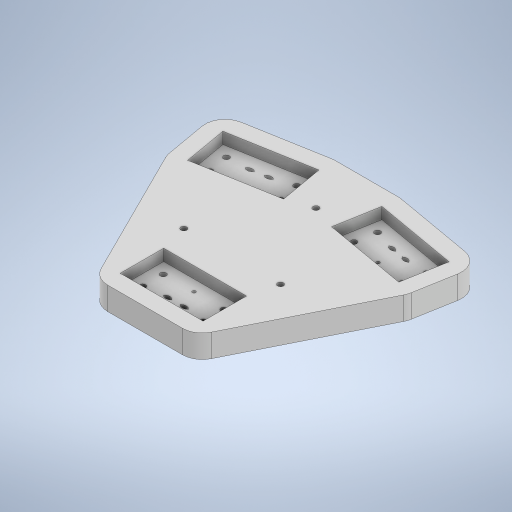
# Autodesk Inventor part: Baseplate
Saved by Autodesk Inventor 2023 (Build 270158000, 158)
## iProperties
Created: 2023-07-20
Part Number: Baseplate
Material: Generic
Document SubType Name: Modeling
Designer: campstudent
Density: 1 g/cm^3
Appearance: Default
Author: campstudent
Autodesk Inventor part; units mm, degrees
ref_plane "YZ Plane" through (0, 0, 0) normal (1, 0, 0) x (0, 1, 0)
ref_plane "XZ Plane" through (0, 0, 0) normal (0, 1, 0) x (-1, 0, 0)
ref_plane "XY Plane" through (0, 0, 0) normal (0, 0, 1) x (1, 0, 0)
sketch "Sketch1" plane through (0, 0, 0) normal (0, 1, 0) x (-1, 0, 0)
  line L0 (0, 0) -> (-160, 0)
  line L1 (-160, 0) -> (-160, -160)
  line L2 (-160, -160) -> (0, -160)
  line L3 (0, -160) -> (0, 0)
  dimension "d0" = 160
  dimension "d1" = 160
  constraints: 8 end point, 2 parallel, 1 horizontal, 1 perpendicular
  measures "d0" distance of L2.end L0.start
  measures "d1" distance of L0.end L0.start
extrude "Extrusion1" add sketch "Sketch1" along normal blind 14
sketch "Sketch2" plane through (0, 14, 0) normal (0, 1, 0) x (1, 0, 0)
  line L0 (54.75, 30) -> (105.25, 30)
  line L1 (105.25, 30) -> (105.25, 56.5)
  line L2 (105.25, 56.5) -> (54.75, 56.5)
  line L3 (54.75, 56.5) -> (54.75, 30)
  line L4 (0, 0) -> (160, 0) projected
  line L5 (0, 160) -> (0, 0) projected
  line L6 (11.0918, 136.251) -> (15.6934, 110.1536)
  line L7 (15.6934, 110.1536) -> (65.4262, 118.9228)
  line L8 (65.4262, 118.9228) -> (60.8246, 145.0203)
  line L9 (60.8246, 145.0203) -> (11.0918, 136.251)
  line L10 (38.2588, 94.75) -> (38.2588, 145.25) construction
  line L11 (25.009, 127.5869) -> (51.509, 127.5869) construction
  line L12 (160, 160) -> (0, 160) projected
  line L13 (54.75, 43.25) -> (106.8484, 43.25) construction
  line L14 (80, 30) -> (80, 56.5) construction
  line L15 (80, 43.25) -> (80, 148.25)
  line L16 (148.9082, 136.251) -> (144.3066, 110.1536)
  line L17 (144.3066, 110.1536) -> (94.5738, 118.9228)
  line L18 (94.5738, 118.9228) -> (99.1754, 145.0203)
  line L19 (99.1754, 145.0203) -> (148.9082, 136.251)
  line L20 (98.0138, 136.2229) -> (145.4682, 118.9509) construction
  line L21 (126.2728, 140.0379) -> (117.2092, 115.136) construction
  line L22 (121.741, 127.5869) -> (85.8289, 28.9192)
  line L23 (38.259, 127.5869) -> (56.4995, 24.14) construction
  point P0 (38.2588, 120)
  point P1 (33.7272, 140.0379)
  point P2 (61.9862, 136.2229)
  dimension "d4" = 26.5
  dimension "d5" = 50.5
  dimension "d6" = 30
  dimension "d7" = 80
  dimension "d9" = 27.167
  dimension "d13" = 17.4333
  dimension "d15" = 12.4509
  dimension "d16" = 23.7272
  dimension "d17" = 11.0918
  dimension "d19" = 105
  dimension "d73" = 270
  constraints: 42 end point, 7 midpoint, 4 parallel, 2 equal length, 2 horizontal, 2 perpendicular, 2 point on line
  measures "d4" distance of L2.end L0.start
  measures "d5" distance of L0.start L0.end
  measures "d6" distance from line of L4 L0.start
  measures "d7" distance from line of L14.start L5
  measures "d9" horizontal distance of L6.start point (38.259, 120)
  measures "d13" vertical distance of L23.start L6.end
  measures "d15" vertical distance of L23.start point (33.727, 140.038)
  measures "d16" horizontal distance of point (61.986, 136.223) L23.start
  measures "d17" horizontal distance of L5.start L6.start
  measures "d19" distance of L15.start L15.end
extrude "Extrusion2" cut sketch "Sketch2" against normal blind 7
sketch "Sketch3" plane through (0, 7, 0) normal (0, 1, 0) x (1, 0, 0)
  circle A0 centre (21.1254, 118.2194) radius 1.8
  line L0 (11.0918, 136.251) -> (60.8246, 145.0203) construction
  line L1 (35.9582, 140.6356) -> (40.5598, 114.5382) construction
  line L2 (65.4262, 118.9228) -> (15.6934, 110.1536) construction
  circle A1 centre (18.9548, 130.5295) radius 1.8
  line L3 (15.6934, 110.1536) -> (11.0918, 136.251) projected
  circle A2 centre (57.5633, 124.6444) radius 1.8
  circle A3 centre (55.3926, 136.9545) radius 1.8
  line L4 (160, 160) -> (0, 160) construction
  line L5 (80, 160) -> (80, 0) construction
  line L6 (0, 0) -> (160, 0) construction
  circle A4 centre (138.8746, 118.2194) radius 1.8
  line L7 (124.0418, 140.6356) -> (119.4402, 114.5382) construction
  circle A5 centre (141.0452, 130.5295) radius 1.8
  circle A6 centre (102.4367, 124.6444) radius 1.8
  circle A7 centre (104.6074, 136.9545) radius 1.8
  circle A8 centre (61.5, 37) radius 1.8
  circle A9 centre (61.5, 49.5) radius 1.8
  line L8 (54.75, 56.5) -> (105.25, 56.5) projected
  line L9 (54.75, 30) -> (54.75, 56.5) projected
  line L10 (105.25, 30) -> (54.75, 30) projected
  circle A10 centre (98.5, 37) radius 1.8
  circle A11 centre (98.5, 49.5) radius 1.8
  circle A12 centre (120.6123, 121.1857) radius 1
  line L11 (144.3066, 110.1536) -> (94.5738, 118.9228) projected
  circle A13 centre (127.4464, 131.1503) radius 1.25
  line L12 (148.9082, 136.251) -> (144.3066, 110.1536) projected
  line L13 (127.4464, 131.1503) -> (129.9085, 130.7162) construction
  line L14 (129.9085, 130.7162) -> (124.9844, 131.5845) construction
  line L15 (99.1754, 145.0203) -> (148.9082, 136.251) construction
  arc A14 (129.9085, 130.7162) -> (124.9844, 131.5845) centre (127.1209, 129.3038) ccw
  arc A15 (124.9844, 131.5845) -> (129.9085, 130.7162) centre (127.772, 132.9968) ccw
  circle A16 centre (117.5984, 132.8868) radius 1.25
  line L16 (117.5984, 132.8868) -> (115.1364, 133.3209) construction
  line L17 (115.1364, 133.3209) -> (120.0604, 132.4527) construction
  arc A17 (120.0604, 132.4527) -> (115.1364, 133.3209) centre (117.2728, 131.0403) ccw
  arc A18 (115.1364, 133.3209) -> (120.0604, 132.4527) centre (117.924, 134.7333) ccw
  circle A19 centre (39.3877, 121.1857) radius 1
  circle A20 centre (32.5536, 131.1503) radius 1.25
  line L18 (32.5536, 131.1503) -> (30.0915, 130.7162) construction
  line L19 (30.0915, 130.7162) -> (35.0156, 131.5845) construction
  arc A21 (35.0156, 131.5845) -> (30.0915, 130.7162) centre (32.8791, 129.3038) ccw
  arc A22 (30.0915, 130.7162) -> (35.0156, 131.5845) centre (32.228, 132.9968) ccw
  line L20 (42.4016, 132.8868) -> (44.8636, 133.3209) construction
  circle A23 centre (42.4016, 132.8868) radius 1.25
  line L21 (44.8636, 133.3209) -> (39.9396, 132.4527) construction
  arc A24 (39.9396, 132.4527) -> (44.8636, 133.3209) centre (42.076, 134.7333) ccw
  arc A25 (44.8636, 133.3209) -> (39.9396, 132.4527) centre (42.7272, 131.0403) ccw
  circle A26 centre (80, 49.75) radius 1
  circle A27 centre (85, 38.75) radius 1.25
  line L22 (105.25, 56.5) -> (105.25, 30) projected
  line L23 (85, 38.75) -> (87.5, 38.75) construction
  line L24 (87.5, 38.75) -> (82.5, 38.75) construction
  arc A28 (82.5, 38.75) -> (87.5, 38.75) centre (85, 40.625) ccw
  arc A29 (87.5, 38.75) -> (82.5, 38.75) centre (85, 36.875) ccw
  circle A30 centre (75, 38.75) radius 1.25
  line L25 (75, 38.75) -> (72.5, 38.75) construction
  line L26 (72.5, 38.75) -> (77.5, 38.75) construction
  arc A31 (72.5, 38.75) -> (77.5, 38.75) centre (75, 40.625) ccw
  arc A32 (77.5, 38.75) -> (72.5, 38.75) centre (75, 36.875) ccw
  line L27 (54.75, 43.25) -> (105.25, 43.25) construction
  line L28 (105.25, 56.5) -> (105.25, 30) construction
  line L29 (146.6074, 123.2023) -> (96.8746, 131.9716) construction
  line L30 (94.5738, 118.9228) -> (99.1754, 145.0203) construction
  point P0 (80, 59.75)
  point P1 (80, 69.75)
  point P2 (127.4464, 131.1503)
  dimension "d24" = 3.6
  dimension "d25" = 7
  dimension "d26" = 6.75
  dimension "d27" = 6.75
  dimension "d28" = 7
  dimension "d29" = 7
  dimension "d30" = 6.75
  dimension "d31" = 3.6
  dimension "d32" = 6.75
  dimension "d33" = 7
  dimension "d36" = 2
  dimension "d37" = 6.75
  dimension "d38" = 2.5
  dimension "d39" = 20.25
  dimension "d41" = 2.5
  dimension "d42" = 2.5
  dimension "d43" = 2
  dimension "d44" = 6.75
  dimension "d45" = 2.5
  dimension "d46" = 20.25
  dimension "d48" = 2.5
  dimension "d49" = 2.5
  dimension "d74" = 10
  dimension "d75" = 10
  dimension "d79" = 4.5
  dimension "d80" = 4.5
  constraints: 34 end point, 33 centre point, 33 symmetric about line, 24 point on circle, 10 midpoint, 10 point on line, 4 tangent, 2 equal radius, 2 perpendicular, 21 other
  measures "d24" diameter of A0
  measures "d25" distance from line of L2 A0.centre
  measures "d26" distance from line of L3 A0.centre
  measures "d27" distance from line of L3 A1.centre
  measures "d28" distance from line of L0 A1.centre
  measures "d29" distance from line of L8 A9.centre
  measures "d30" distance from line of L9 A9.centre
  measures "d31" diameter of A9
  measures "d32" distance from line of L9 A8.centre
  measures "d33" distance from line of L10 A8.centre
  measures "d36" diameter of A12
  measures "d37" distance from line of L11 A12.centre
  measures "d38" diameter of A13
  measures "d39" distance from line of L12 L13.start
  measures "d41" distance of L14.end L13.start
  measures "d42" distance of L13.end L13.start
  measures "d43" diameter of A26
  measures "d44" distance from line of L8 A26.centre
  measures "d45" diameter of A27
  measures "d46" distance from line of L22 L23.start
  measures "d48" distance of L23.start L23.end
  measures "d49" distance of L24.end L23.start
  measures "d74" distance of point (80, 59.75) A26.centre
  measures "d75" distance of point (80, 69.75) point (80, 59.75)
  measures "d79" distance from line of L27 point (85, 38.75)
  measures "d80" distance from line of L29 point (127.446, 131.15)
extrude "Extrusion3" cut sketch "Sketch3" against normal blind 7 contours A0 | A1 | A2 | A3 | A4 | A5 | A6 | A7 | A8 | A9 | A10 | A11 | A12 | A13 | A13 A14 A15 | A13 A15 A14 | A16 | A16 A17 A18 | A16 A18 A17 | A19 | A20 | A20 A21 A22 | A20 A22 A21 | A23 | A23 A25 A24 | A23 A24 A25 | A26 | A27 | A27 A29 A28 | A27 A28 A29 | A30 | A30 A32 A31 | A30 A31 A32
sketch "Sketch5" plane through (0, 14, 0) normal (0, 1, 0) x (1, 0, 0)
  line L0 (0, 160) -> (0, 0) projected
  line L1 (0, 144.4495) -> (88.1912, 160)
  line L2 (160, 160) -> (0, 160) projected
  line L3 (71.8088, 160) -> (160, 144.4495)
  line L4 (160, 0) -> (160, 160) projected
  line L5 (11.0918, 136.251) -> (60.8246, 145.0203) projected
  line L6 (99.1754, 145.0203) -> (148.9082, 136.251) projected
  line L7 (0, 120) -> (59.75, 0)
  line L8 (0, 0) -> (160, 0) projected
  line L9 (160, 120) -> (100.25, 0)
  line L10 (54.75, 30) -> (54.75, 56.5) projected
  line L11 (105.25, 56.5) -> (105.25, 30) projected
  line L12 (0, 144.4495) -> (0, 160)
  line L13 (88.1912, 160) -> (0, 160)
  line L14 (160, 144.4495) -> (160, 160)
  line L15 (71.8088, 160) -> (160, 160)
  line L16 (160, 0) -> (160, 120)
  line L17 (100.25, 0) -> (160, 0)
  line L18 (0, 120) -> (0, 0)
  line L19 (0, 0) -> (59.75, 0)
  line L20 (49.7917, 20) -> (110.2083, 20)
  line L21 (105.25, 30) -> (54.75, 30) projected
  line L22 (160, 144.4495) -> (134.5297, 0)
  line L23 (0, 0) -> (160, 0) projected
  line L24 (148.9082, 136.251) -> (144.3066, 110.1536) projected
  line L25 (0, 144.4495) -> (25.4703, 0)
  line L26 (15.6934, 110.1536) -> (11.0918, 136.251) projected
  line L27 (0, 160) -> (0, 0) projected
  line L28 (0, 155) -> (160, 155)
  point P0 (115.9044, 152.2248)
  point P1 (100.25, 0)
  point P2 (71.8088, 160)
  point P3 (153.3251, 106.5944)
  point P4 (6.6749, 106.5944)
  point P5 (59.8348, 155)
  point P6 (100.1652, 155)
  point P7 (80, 158.5557)
  dimension "d50" = 10
  dimension "d51" = 10
  dimension "d52" = 120
  dimension "d54" = 120
  dimension "d56" = 5
  dimension "d57" = 5
  dimension "d60" = 10
  dimension "d78" = 5
  constraints: 32 end point, 12 point on line, 4 collinear, 4 parallel, 2 equal length, 2 horizontal, 1 midpoint, 1 perpendicular
  measures "d50" distance between parallel lines of L5 L1
  measures "d51" distance from line of L6 point (115.904, 152.225)
  measures "d52" distance of L0.end L7.start
  measures "d54" distance of L4.start L9.start
  measures "d56" distance from line of L10 L7.end
  measures "d57" distance from line of L9.end L11
  measures "d60" distance between parallel lines of L20 L21
  measures "d78" distance between parallel lines of L2 L28
extrude "Extrusion4" cut sketch "Sketch5" against normal through all contours L2 L3 L1 L28 L0 | L28 L1 L0 | L2 L1 L3 | L25 L7 L0 | L1 L3 L28 | L2 L4 L28 L3 L1 | L7 L25 L8 L0 | L7 L8 L25 | L28 L4 L3 | L20 L9 L8 L7 | L4 L9 L22 | L9 L22 L8 | L4 L8 L22 L9
fillet "Fillet1" radius 12 8 edges at (110.2083, 7, -20) (49.7917, 7, -20) (0, 7, -144.4495) (6.6749, 7, -106.5944) (59.8348, 7, -155) (100.1652, 7, -155) (160, 7, -144.4495) (153.3251, 7, -106.5944)
sketch "Sketch6" plane through (0, 14, 0) normal (0, 1, 0) x (1, 0, 0)
  circle A0 centre (80, 90) radius 34
  line L0 (99.96, 160) -> (60.04, 160) projected
  line L1 (160, 120.9408) -> (160, 141.0931) projected
  line L2 (80, 90) -> (80, 18.0727) construction
  line L3 (80, 90) -> (28.0347, 59.9978) construction
  line L4 (80, 90) -> (140.0044, 90) construction
  circle A1 centre (50.5551, 73) radius 1.8
  circle A2 centre (109.4449, 73) radius 1.8
  circle A3 centre (80, 124) radius 1.8
  point P0 (0, 0)
  dimension "d62" = 68
  dimension "d63" = 70
  dimension "d64" = 80
  dimension "d65" = 150
  dimension "d66" = 3.6
  dimension "d69" = 360
  constraints: 6 end point, 3 centre point, 1 equal length, 1 horizontal, 1 point on line, 1 vertical, 10 other
  measures "d63" distance from line of L2.start L0
  measures "d64" distance from line of L1 L2.start
  measures "d65" angle of L3 L4
  measures "d66" diameter of A1
extrude "Extrusion5" cut sketch "Sketch6" against normal through all contours A3 A0 | A0 A3 | A2 A0 | A0 A2 | A1 A0 | A0 A1
body "Solid1"
